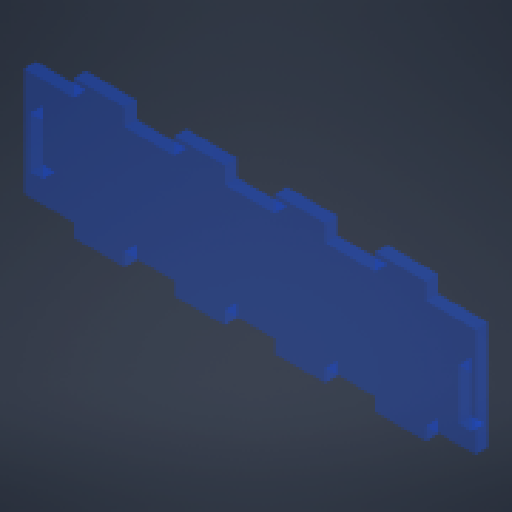
# Autodesk Inventor part: Acrilico-Parachoque-Parede-Inf
Saved by Autodesk Inventor 2026 (Build 300175000, 175)
## iProperties
Created: 2025-09-30
Part Number: Acrilico-Parachoque-Parede-Inf
Material: Genérico
Document SubType Name: Modeling
Designer: Nitro
Density: 1 g/cm^3
Appearance: Transparente - Azul
Author: Nitro
Autodesk Inventor part; units mm, degrees
ref_plane "YZ Plane" through (0, 0, 0) normal (1, 0, 0) x (0, 1, 0)
ref_plane "XZ Plane" through (0, 0, 0) normal (0, 1, 0) x (-1, 0, 0)
ref_plane "XY Plane" through (0, 0, 0) normal (0, 0, 1) x (1, 0, 0)
sketch "Esboço1" plane through (0, 0, 0) normal (0, 0, 1) x (1, 0, 0)
  line L0 (-55, 14.75) -> (52, 14.75)
  line L1 (52, 14.75) -> (52, -18)
  line L2 (52, -18) -> (-55, -18)
  line L3 (-55, -18) -> (-55, 14.75)
  line L4 (52.0001, 13.75) -> (52.0001, 10.75) projected
  line L5 (-50.5, -18) -> (-53.5, -18)
  point P0 (0, 0)
  dimension "d34" = 52
  dimension "d35" = 18
  dimension "d36" = 14.75
  constraints: 10 end point, 2 horizontal, 2 parallel, 1 perpendicular, 2 other
  measures "d34" distance from line of L1 point (0, 0)
  measures "d35" distance from line of L2 point (0, 0)
  measures "d36" distance from line of L0 point (0, 0)
extrude "Extrusão1" add sketch "Esboço1" along normal blind 3
sketch "Esboço2" plane through (0, 0, 3) normal (0, 0, 1) x (1, 0, 0)
  line L0 (19.2209, 13.75) -> (19.2209, 10.75) projected
  line L1 (52, 14.75) -> (-55, 14.75) projected
  line L2 (-55, 14.75) -> (-55, -18) projected
  line L3 (-55, 14.75) -> (-43.2, 14.75)
  line L4 (-43.2, 14.75) -> (-43.2, 10.75)
  line L5 (-43.2, 10.75) -> (-55, 10.75)
  line L6 (-55, 10.75) -> (-55, 14.75)
  line L7 (-19.4, 14.75) -> (-19.4, 10.75)
  line L8 (-19.4, 10.75) -> (-31.2, 10.75)
  line L9 (-31.2, 10.75) -> (-31.2, 14.75)
  line L10 (-31.2, 14.75) -> (-19.4, 14.75)
  line L11 (4.4, 14.75) -> (4.4, 10.75)
  line L12 (4.4, 10.75) -> (-7.4, 10.75)
  line L13 (-7.4, 10.75) -> (-7.4, 14.75)
  line L14 (-7.4, 14.75) -> (4.4, 14.75)
  line L15 (28.2, 14.75) -> (28.2, 10.75)
  line L16 (28.2, 10.75) -> (16.4, 10.75)
  line L17 (16.4, 10.75) -> (16.4, 14.75)
  line L18 (16.4, 14.75) -> (28.2, 14.75)
  line L19 (-55, -18) -> (-43.2, -18)
  line L20 (-43.2, -18) -> (-43.2, -14.869)
  line L21 (-43.2, -14.869) -> (-55, -14.869)
  line L22 (-55, -14.869) -> (-55, -18)
  line L23 (-19.4, -18) -> (-19.4, -14.869)
  line L24 (-31.2, -18) -> (-19.4, -18)
  line L25 (-31.2, -14.869) -> (-31.2, -18)
  line L26 (-19.4, -14.869) -> (-31.2, -14.869)
  line L27 (4.4, -18) -> (4.4, -14.869)
  line L28 (-7.4, -18) -> (4.4, -18)
  line L29 (-7.4, -14.869) -> (-7.4, -18)
  line L30 (4.4, -14.869) -> (-7.4, -14.869)
  line L31 (28.2, -18) -> (28.2, -14.869)
  line L32 (16.4, -18) -> (28.2, -18)
  line L33 (16.4, -14.869) -> (16.4, -18)
  line L34 (28.2, -14.869) -> (16.4, -14.869)
  line L35 (52, -18) -> (52, -14.869)
  line L36 (40.2, -18) -> (52, -18)
  line L37 (40.2, -14.869) -> (40.2, -18)
  line L38 (52, -14.869) -> (40.2, -14.869)
  line L39 (-53.4999, 2.375) -> (-50.4999, 2.375) projected
  line L40 (-50.4999, 2.375) -> (-50.4999, -9.625) projected
  line L41 (-50.4999, -9.625) -> (-53.4999, -9.625) projected
  line L42 (-53.4999, 2.375) -> (-53.4999, -9.625) projected
  line L43 (-53.4999, -9.625) -> (-50.4999, -9.625)
  line L44 (-50.4999, -9.625) -> (-50.4999, 2.375)
  line L45 (-50.4999, 2.375) -> (-53.4999, 2.375)
  line L46 (-53.4999, 2.375) -> (-53.4999, -9.625)
  line L47 (52, 14.75) -> (52, 10.75)
  line L48 (52, 10.75) -> (40.2, 10.75)
  line L49 (40.2, 10.75) -> (40.2, 14.75)
  line L50 (40.2, 14.75) -> (52, 14.75)
  line L51 (51, 5.506) -> (48, 5.506) projected
  line L52 (48, 5.506) -> (48, -6.494) projected
  line L53 (48, -6.494) -> (51, -6.494) projected
  line L54 (51, 5.506) -> (51, -6.494) projected
  line L55 (48, 5.506) -> (51, 5.506)
  line L56 (51, 5.506) -> (51, -6.494)
  line L57 (51, -6.494) -> (48, -6.494)
  line L58 (48, -6.494) -> (48, 5.506)
  point P0 (52, -18)
  point P1 (4.4, 14.75)
  point P2 (-43.2, 14.75)
  dimension "d37" = 11.8
  dimension "d38" = 4
  dimension "d41" = 23.8
  dimension "d46" = 11.8
  dimension "d49" = 23.8
  constraints: 96 end point, 8 parallel, 6 horizontal, 4 perpendicular, 64 other
  measures "d37" distance of L4.end L5.end
  measures "d38" distance of L3.end L4.end
  measures "d41" distance of L4.end L7.end
  measures "d46" distance of L21.end L20.end
  measures "d49" distance of L20.end L23.end
extrude "Extrusão2" cut sketch "Esboço2" against normal through all
